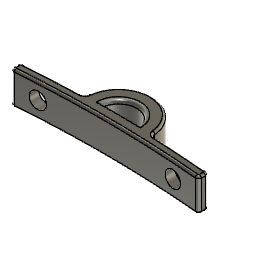
phalanx guide straight (Autodesk Fusion 360 design; units mm, degrees)
Autodesk Fusion 360 part; units mm, degrees
note: some values were not read from the file. Chosen so that the rebuilt part matches the saved one: that a step has no effect.
sketch "Sketch1" plane through (0, 0, 0) normal (0, 0, 1) x (1, 0, 0)
  arc A0 (2.2398, 0.2139) -> (-2.2372, 0.24) centre (0, 0) ccw
  arc A1 (1.2499, -0.0177) -> (-1.25, -0.0031) centre (0, 0) ccw
  line L0 (-6.3742, -0.419) -> (-6.3742, -0.6767)
  line L1 (6.3659, -0.4908) -> (6.3659, -0.7496)
  arc A2 (-75.4331, -74.1986) -> (74.5485, -76.4584) centre (-0.4373, -74.9987) ccw
  arc A3 (6.1483, -0.9489) -> (-6.159, -0.8761) centre (-0.4473, -75.6583) ccw
  arc A4 (-75.4331, -74.1986) -> (74.5485, -76.4584) centre (-0.4473, -75.6583) ccw
  arc A5 (6.3659, -0.4908) -> (6.1835, -0.2915) centre (6.1659, -0.4908) ccw
  arc A6 (6.1483, -0.9489) -> (6.3659, -0.7496) centre (6.1659, -0.7496) ccw
  arc A7 (-6.3742, -0.6767) -> (-6.159, -0.8761) centre (-6.1742, -0.6767) ccw
  arc A8 (-6.19, -0.2197) -> (-6.3742, -0.419) centre (-6.1742, -0.419) ccw
  arc A9 (6.1835, -0.2915) -> (2.5266, -0.0573) centre (-0.4373, -74.9987) ccw
  arc A10 (1.2499, -0.0177) -> (-1.25, -0.0031) centre (-0.4373, -74.9987) ccw
  arc A11 (-2.5271, -0.0278) -> (-6.19, -0.2197) centre (-0.4373, -74.9987) ccw
  arc A12 (2.2398, 0.2139) -> (2.5266, -0.0573) centre (2.5384, 0.2425) ccw
  arc A13 (-2.5271, -0.0278) -> (-2.2372, 0.24) centre (-2.5354, 0.272) ccw
  dimension "d1" = 4.5
  dimension "d2" = 2.5
  dimension "d3" = 150
  dimension "d4" = 150
  dimension "d5" = 0.2
  dimension "d6" = 0.3
  constraint coincident A0.centre A1.centre
  constraint coincident A0.centre A9
  constraint coincident A1.end A9
  constraint coincident A1.start A9
  constraint vertical L0
  constraint vertical L1
  constraint coincident A2.start A3
  constraint concentric A2 A9
  constraint concentric A3 A4
  constraint tangent A5 A9
  constraint tangent L1 A5
  constraint tangent A3 A6
  constraint tangent L1 A6
  constraint equal A5 A6
  constraint tangent L0 A7
  constraint tangent A3 A7
  constraint equal A5 A7
  constraint tangent A8 A9
  constraint tangent L0 A8
  constraint equal A5 A8
  constraint concentric A9 A10
  constraint concentric A10 A11
  constraint tangent A0 A12
  constraint tangent A9 A12
  constraint tangent A0 A13
  constraint tangent A11 A13
  constraint equal A12 A13
  measures "d1" diameter of A0
  measures "d2" diameter of A1
  measures "d3" diameter of A9
  measures "d4" diameter of A3
  measures "d5" radius of A5
  measures "d6" radius of A12
extrude "Extrude1" add sketch "Sketch1" along normal blind 2.2 contours A0 L0 L1 A3 A5 A6 A7 A8 A9 A11 A12 A13
fillet "Fillet1" [no effect]
sketch "Sketch2" plane through (0, 0, 0) normal (0, 1, 0) x (1, 0, 0)
  circle A0 centre (4.5, -1.1) radius 0.55
  circle A1 centre (-4.6757, -1.1) radius 0.55
  line L0 (-6.19, -2.2) -> (-2.5271, -2.2)
  line L1 (2.5266, -2.2) -> (6.1835, -2.2)
  dimension "d13" = 1.1
  dimension "d14" = 1.1
  dimension "d16" = 1.1
  dimension "d17" = 1.1
  measures "d13" diameter of A0
  measures "d14" diameter of A1
  measures "d16" distance of A1.centre L0
  measures "d17" distance of A0.centre L1
extrude "Extrude2" cut sketch "Sketch2" against normal blind 1
fillet "Fillet2" radius 0.25 3 edges at (0.0073, 1.25, 0) (0.0073, 1.25, 2.2) (0, 0, 0)
fillet "Fillet3" radius 0.1 12 edges at (-6.3101, -0.8234, 0) (-6.3742, -0.5479, 0) (-6.3211, -0.2833, 0) (-4.3597, -0.1014, 0) (-2.3319, 0.0517, 0) (0.0131, 2.25, 0) (2.3323, 0.0245, 0) (4.3565, -0.1521, 0) (6.3134, -0.3557, 0) (6.3659, -0.6202, 0) (6.3009, -0.8971, 0) (-0.0039, -0.6596, 0)
fillet "Fillet4" radius 0.15 12 edges at (0.0131, 2.25, 2.2) (-2.3319, 0.0517, 2.2) (-4.3597, -0.1014, 2.2) (-6.3211, -0.2833, 2.2) (-6.3742, -0.5479, 2.2) (-6.3101, -0.8234, 2.2) (-0.0039, -0.6596, 2.2) (6.3009, -0.8971, 2.2) (6.3659, -0.6202, 2.2) (6.3134, -0.3557, 2.2) (4.3565, -0.1521, 2.2) (2.3323, 0.0245, 2.2)
